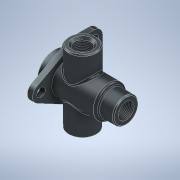
# Autodesk Inventor part: 1-阀体
Saved by Autodesk Inventor 2022 (Build 260153000, 153)
## iProperties
Created: 2023-01-24
Part Number: 1-阀体
Material: 灰口铁
Document SubType Name: Modeling
Designer: Lzy18
Density: 7.15 g/cm^3
Appearance: 灰口铁
Author: Lzy18
Autodesk Inventor part; units mm, degrees
ref_plane "YZ Plane" through (0, 0, 0) normal (1, 0, 0) x (0, 1, 0)
ref_plane "XZ Plane" through (0, 0, 0) normal (0, 1, 0) x (-1, 0, 0)
ref_plane "XY Plane" through (0, 0, 0) normal (0, 0, 1) x (1, 0, 0)
sketch "草图1" plane through (0, 0, 0) normal (0, 0, 1) x (1, 0, 0)
  line L0 (-13, 34) -> (13, 34)
  line L1 (13, 34) -> (13, -34)
  line L2 (13, -34) -> (-13, -34)
  line L3 (-13, -34) -> (-13, 34)
  line L4 (-13, 34) -> (13, -34) construction
  line L5 (13, 34) -> (-13, -34) construction
  line L6 (0, 34) -> (0, -34)
  point P0 (0, 0)
  dimension "d0" = 26
  dimension "d1" = 68
  constraints: 14 end point, 4 midpoint, 2 parallel, 1 horizontal, 1 perpendicular
  measures "d0" distance of L1.end L2.end
  measures "d1" distance of L0.end L1.end
revolve "旋转1" add sketch "草图1" angle 360 about axis through (0, 34, 0) along (0, -1, 0) contours L0 L1 L2 L6
sketch "草图2" plane through (0, 0, 0) normal (1, 0, 0) x (0, 1, 0)
  circle A0 centre (0, 0) radius 15
  dimension "d3" = 30
  constraints: 1 centre point, 1 coincident
  measures "d3" diameter of A0
extrude "拉伸1" add sketch "草图2" along normal blind 27
sketch "草图3" plane through (27, 0, 0) normal (1, 0, 0) x (0, 0, -1)
  circle A0 centre (0, 0) radius 12
  dimension "d6" = 24
  constraints: 1 centre point, 1 coincident
  measures "d6" diameter of A0
extrude "拉伸2" add sketch "草图3" along normal blind 14
sketch "草图4" plane through (0, 0, 0) normal (1, 0, 0) x (0, 1, 0)
  circle A0 centre (0, 0) radius 15
  dimension "d9" = 30
  constraints: 1 centre point, 1 coincident
  measures "d9" diameter of A0
extrude "拉伸3" add sketch "草图4" against normal blind 14
sketch "草图5" plane through (-14, 0, 0) normal (-1, 0, 0) x (0, 0, 1)
  line L0 (-2.5, 26) -> (-25, 26)
  line L1 (-33, 18) -> (-33, -18)
  line L2 (-25, -26) -> (-2.5, -26)
  circle A0 centre (-25, 18) radius 4
  line L3 (0, 0) -> (-33, 0)
  circle A1 centre (-25, -18) radius 4
  arc A2 (0, 23.5) -> (-2.5, 26) centre (-2.5, 23.5) ccw
  arc A3 (0, 23.5) -> (1.0638, 21.7327) centre (2, 23.5) ccw
  arc A4 (28.7448, -7.0694) -> (28.7448, 7.0694) centre (25, 0) ccw
  circle A5 centre (25, 0) radius 4
  line L4 (1.0638, 21.7327) -> (28.7448, 7.0694)
  arc A6 (-2.5, -26) -> (0, -23.5) centre (-2.5, -23.5) ccw
  arc A7 (1.0638, -21.7327) -> (0, -23.5) centre (2, -23.5) ccw
  line L5 (1.0638, -21.7327) -> (28.7448, -7.0694)
  arc A8 (-25, 26) -> (-33, 18) centre (-25, 18) ccw
  arc A9 (-33, -18) -> (-25, -26) centre (-25, -18) ccw
  point P0 (-0.7322, 25.2678)
  dimension "d16" = 8
  dimension "d21" = 50
  constraints: 15 point on circle, 12 end point, 10 centre point, 10 symmetric about line, 4 tangent, 2 coincident, 2 perpendicular, 1 midpoint, 7 other
  measures "d16" distance from line of L0 A0.centre
  measures "d21" horizontal distance of A0.centre A4.centre
extrude "拉伸4" add sketch "草图5" along normal blind 5
sketch "草图6" plane through (-19, 0, 0) normal (-1, 0, 0) x (0, 0, 1)
  circle A0 centre (0, 0) radius 16.5
  dimension "d25" = 33
  constraints: 1 centre point, 1 coincident
  measures "d25" diameter of A0
extrude "拉伸5" add sketch "草图6" along normal blind 8
sketch "草图7" plane through (-27, 0, 0) normal (-1, 0, 0) x (0, 0, 1)
  circle A0 centre (0, 0) radius 16.5 projected
  constraints: 1 coincident
hole "孔1" at (-27, 0, 0) direction (1, 0, 0) diameter 23.752 depth 12 thread size "M27x3" designation "M27" class "6H" standard "GB Metric profile"
sketch "草图8" plane through (0, 34, 0) normal (0, 1, 0) x (1, 0, 0)
  circle A0 centre (0, 0) radius 13 projected
  constraints: 1 coincident
hole "孔2" at (0, 34, 0) direction (0, -1, 0) diameter 14.95 depth 14 thread size "G16.662x1.337" designation "G 3/8" standard "GB Pipe Threads without seal"
sketch "草图9" plane through (0, 0, 0) normal (0, 0, 1) x (1, 0, 0)
  line L0 (0, 15) -> (0, 20)
  line L1 (0, -47.6) -> (0, 47.6) projected
  line L2 (0, 15) -> (-5, 15)
  line L3 (-5, 15) -> (-7.8868, 20)
  line L4 (0, 20) -> (-7.8868, 20)
  line L5 (7.475, 20) -> (-7.475, 20) projected
  point P0 (0, 0)
  point P1 (0, 17.5)
  dimension "d68" = 5
  dimension "d69" = 30
  constraints: 8 end point, 1 collinear, 1 horizontal, 1 midpoint, 1 other
  measures "d68" distance of L0.start L2.end
  measures "d69" angle of L3 L0
revolve "旋转2" cut sketch "草图9" angle 360 about axis through (0, -10, 0) along (0, 1, 0)
sketch "草图10" plane through (41, 0, 0) normal (1, 0, 0) x (0, 0, -1)
  circle A0 centre (0, 0) radius 12 projected
  constraints: 1 coincident
hole "孔3" at (41, 0, 0) direction (-1, 0, 0) diameter 14.95 depth 14 thread size "G16.662x1.337" designation "G 3/8" standard "GB Pipe Threads without seal"
sketch "草图11" plane through (0, 0, 0) normal (0, 0, 1) x (1, 0, 0)
  line L0 (27, -15) -> (27, 15) projected
  line L1 (27, 0) -> (22, 0)
  line L2 (27, -7.475) -> (27, 7.475) projected
  line L3 (27, 0) -> (27, 7.475)
  line L4 (-40.6, 0) -> (54.6, 0) projected
  line L5 (22, 0) -> (22, 5)
  line L6 (22, 5) -> (27, 7.8868)
  line L7 (27, 7.8868) -> (27, 0)
  point P0 (0, 0)
  dimension "d54" = 5
  dimension "d70" = 5
  dimension "d71" = 30
  constraints: 10 end point, 2 collinear, 1 horizontal, 1 midpoint, 1 point on line, 1 vertical
  measures "d54" distance of L1.start L1.end
  measures "d70" distance of L1.end L5.end
  measures "d71" angle of L6 L1
revolve "旋转3" cut sketch "草图11" angle 360 about axis through (-10, 0, 0) along (1, 0, 0)
sketch "草图12" plane through (-15, 0, 0) normal (-1, 0, 0) x (0, 0, 1)
  circle A0 centre (0, 0) radius 11.876 projected
  constraints: 1 coincident
hole "孔4" at (-15, 0, 0) direction (1, 0, 0) diameter 29 depth 2
sketch "草图15" plane through (22, 0, 0) normal (1, 0, 0) x (0, 0, -1)
  circle A0 centre (0, 0) radius 5 projected
  constraints: 1 coincident
hole "孔6" at (22, 0, 0) direction (-1, 0, 0) diameter 10 end through all
sketch "草图16" plane through (0, -34, 0) normal (0, -1, 0) x (1, 0, 0)
  circle A0 centre (0, 0) radius 13 projected
  constraints: 1 coincident
hole "孔7" at (0, -34, 0) direction (0, 1, 0) diameter 14.95 depth 14 thread size "G16.662x1.337" designation "G 3/8" standard "GB Pipe Threads without seal"
sketch "草图17" plane through (0, 0, 0) normal (0, 0, 1) x (1, 0, 0)
  line L0 (-7.475, -20) -> (7.475, -20) projected
  line L1 (0, -20) -> (0, -15)
  line L2 (0, -15) -> (5, -15)
  line L3 (5, -15) -> (7.8868, -20)
  line L4 (0, -20) -> (7.8868, -20)
  line L5 (0, -47.6) -> (0, 47.6) projected
  point P0 (0, 0)
  dimension "d96" = 5
  dimension "d97" = 5
  dimension "d98" = 30
  constraints: 8 end point, 1 midpoint, 1 perpendicular, 1 point on line, 1 vertical
  measures "d96" distance of L1.start L1.end
  measures "d97" distance of L1.end L2.end
  measures "d98" angle of L1 L3
revolve "旋转5" cut sketch "草图17" angle 360 about axis through (0, -10, 0) along (0, 1, 0)
chamfer "倒角5" distance 1 angle 45 4 edges at (-27, 0, -16.5) (-13, 34, 0) (-13, -34, 0) (41, 0, 12)
chamfer "倒角6" distance 2 angle 45 2 edges at (0, 34, -7.475) (0, -34, 7.475)
fillet "圆角2" radius 2 9 edges at (-19, 0, -16.5) (8.405, 11.2536, 9.9174) (8.4076, 11.2556, -9.9152) (-8.405, 11.2536, -9.9174) (-8.4077, 11.2556, 9.9152) (8.408, -11.2559, 9.9149) (8.4076, -11.2556, -9.9152) (-13, -15, 0.0018) (27, -15, 0)
fillet "圆角3" radius 1 1 edges at (27, 0, 12)
sketch "草图19" plane through (0, 0, 0) normal (0, 0, 1) x (1, 0, 0)
  line L0 (0, 0) -> (29.5177, 0)
  line L1 (18, 0) -> (18, 8)
  line L2 (22, 5) -> (22, -5) projected
  line L3 (18, 8) -> (-10.5, 10.85)
  line L4 (-10.5, 10.85) -> (-13, 11.1)
  line L5 (-13, 14.5) -> (-13, -14.5) projected
  line L6 (-13, 11.1) -> (-13, 0)
  line L7 (-13, 0) -> (18, 0)
  line L8 (-40.6, 0) -> (54.6, 0) projected
  dimension "d125" = 8
  dimension "d126" = 4
  dimension "d130" = 10.85
  constraints: 12 end point, 3 point on line, 2 vertical, 1 collinear, 1 horizontal
  measures "d125" distance of L1.start L1.end
  measures "d126" distance between parallel lines of L1 L2
  measures "d130" distance from line of L0 L3.end
revolve "旋转6" cut sketch "草图19" angle 360 about axis through (-10, 0, 0) along (1, 0, 0)
sketch "草图21" plane through (0, 15, 0) normal (0, 1, 0) x (1, 0, 0)
  circle A0 centre (0, 0) radius 5 projected
  constraints: 1 coincident
hole "孔9" at (0, 15, 0) direction (0, -1, 0) diameter 10 end through all
